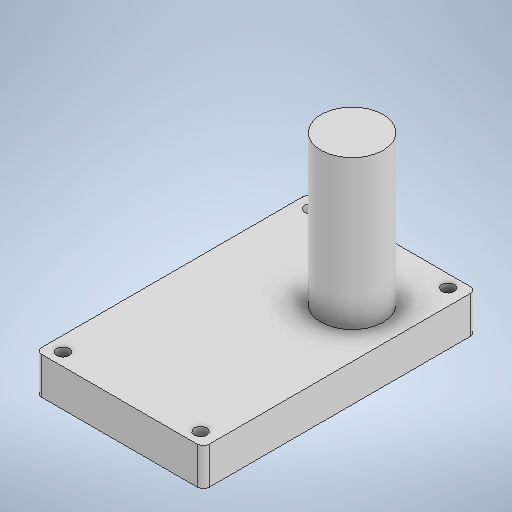
# Autodesk Inventor part: sensor 2
Saved by Autodesk Inventor 2025 (Build 290162000, 162)
## iProperties
Created: 2024-04-10
Part Number: sensor 2
Material: Generic
Document SubType Name: Modeling
Designer: mahal
Density: 1 g/cm^3
Appearance: Default
Author: mahal
Autodesk Inventor part; units mm, degrees
ref_plane "YZ Plane" through (0, 0, 0) normal (1, 0, 0) x (0, 1, 0)
ref_plane "XZ Plane" through (0, 0, 0) normal (0, 1, 0) x (-1, 0, 0)
sketch "Sketch1" plane through (0, 0, 0) normal (0, 1, 0) x (-1, 0, 0)
  line L0 (27, 44) -> (-27, 44)
  line L1 (-27, 44) -> (-27, -44)
  line L2 (-27, -44) -> (27, -44)
  line L3 (27, -44) -> (27, 44)
  line L4 (27, 44) -> (-27, -44) construction
  line L5 (-27, 44) -> (27, -44) construction
  circle A0 centre (22.3059, 39.9545) radius 2
  circle A1 centre (-22.0879, 39.9545) radius 2
  circle A2 centre (-21.9299, -40.0455) radius 2
  circle A3 centre (22.3059, -40.0455) radius 2
  point P0 (0, 0)
  dimension "d0" = 54
  dimension "d6" = 4
  dimension "d7" = 4
  dimension "d8" = 4
  dimension "d9" = 4
  dimension "d17" = 88
  dimension "d19" = 80
  constraints: 12 end point, 4 centre point, 2 midpoint, 2 parallel, 1 horizontal, 1 perpendicular
  measures "d0" distance of L2.end L1.end
  measures "d6" diameter of A0
  measures "d7" diameter of A1
  measures "d8" diameter of A2
  measures "d9" diameter of A3
  measures "d17" distance of L0.end L1.end
  measures "d19" distance of A1.centre A2.centre
extrude "Extrusion1" add sketch "Sketch1" along normal blind 12
ref_plane "Work Plane1" through (0, 12, 0) normal (0, 1, 0) x (1, 0, 0)
sketch "Sketch2" plane through (0, 12, 0) normal (0, 1, 0) x (1, 0, 0)
  circle A0 centre (11, 20) radius 10
  point P0 (0, 0)
  dimension "d14" = 20
  constraints: 1 centre point
  measures "d14" diameter of A0
extrude "Extrusion2" add sketch "Sketch2" along normal blind 48
fillet "Fillet1" radius 2 4 edges at (27, 6, 44) (27, 6, -44) (-27, 6, 44) (-27, 6, -44)
body "Solid1"
